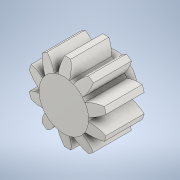
# Autodesk Inventor part: Spur Gear1
Saved by Autodesk Inventor 2022 (Build 260153000, 153)
## iProperties
CustomPartVersion: 1
Created: 2022-03-16
Part Number: Spur Gear1
Material: Steel
Document SubType Name: Modeling
Designer: zac-h
Categories: <?xml version="1.0" encoding="UTF-16"?> <MemberInstance><Categories><FamilyTemplate><FamilyTemplateParameter ValueType="xs:double" Id="1" ObjectReferenceKey="da_z" ObjectType="kUserParameterObject"/><FamilyTemplateParameter ValueType="xs:double" Id="2" ObjectReferenceKey="da_b" ObjectType="kUserParameterObject"/><FamilyTemplateParameter ValueType="xs:double" Id="3" ObjectReferenceKey="da_beta" ObjectType="kUserParameterObject"/><FamilyTemplateParameter ValueType="xs:double" Id="4" ObjectReferenceKey="da_da" ObjectType="kUserParameterObject"/><FamilyTemplateParameter ValueType="xs:double" Id="5" ObjectReferenceKey="da_aw" ObjectType="kUserParameterObject"/><FamilyTemplateParameter ValueType="xs:string" Id="6" ObjectReferenceKey="EAIAABAAAAC/AAAAAAAAAIAAAAAAAAAA" ObjectType="83910656" SubObjectId="SurfaceGeometry"/></FamilyTemplate><ParamToTemplateMap><ParamToTemplate CategoryParameter="//CategoryParameter[@InternalName='046C89C9-8512-4d59-83FE-43B91F4F132A']" TemplateParameter="1"/><ParamToTemplate CategoryParameter="//CategoryParameter[@InternalName='2552DF32-E462-4b46-AEBF-C6C7768E72AC']" TemplateParameter="2"/><ParamToTemplate CategoryParameter="//CategoryParameter[@InternalName='C9EE641D-15FC-4fae-A226-E94C4372FDD7']" TemplateParameter="3"/><ParamToTemplate><ParamToTemplate CategoryParameter="//CategoryParameter[@InternalName='00B6519A-459B-49c7-AD84-2E56D39A5744']" ConstantValue="0.000000"/></ParamToTemplate><ParamToTemplate><ParamToTemplate CategoryParameter="//CategoryParameter[@InternalName='04B31F0E-C7A6-4894-AA32-9629BEFACF47']" ConstantValue="1.000000"/></ParamToTemplate><ParamToTemplate><ParamToTemplate CategoryParameter="//CategoryParameter[@InternalName='43CBEC2E-7847-49e7-A936-2F7889FCB2D9']" ConstantValue="0.250000"/></ParamToTemplate><ParamToTemplate><ParamToTemplate CategoryParameter="//CategoryParameter[@InternalName='B1EFC894-105D-4ebd-86BF-FA20ED196853']" ConstantValue="0.333500"/></ParamToTemplate><ParamToTemplate><ParamToTemplate CategoryParameter="//CategoryParameter[@InternalName='51175063-3D10-4879-93E8-6246FE8B403D']" ConstantValue="2061532430.657340"/></ParamToTemplate><ParamToTemplate><ParamToTemplate CategoryParameter="//CategoryParameter[@InternalName='A3A52E27-4454-46a9-B0BD-C932399B70AF']" ConstantValue="0.300000"/></ParamToTemplate><ParamToTemplate><ParamToTemplate CategoryParameter="//CategoryParameter[@InternalName='91B76062-C214-41d9-B1B9-14D2AB99603D']" ConstantValue="0.100000"/></ParamToTemplate><ParamToTemplate><ParamToTemplate CategoryParameter="//CategoryParameter[@InternalName='374E806E-8B8A-4dda-A9AA-1039D6500AD2']" ConstantValue="10.000000"/></ParamToTemplate><ParamToTemplate><ParamToTemplate CategoryParameter="//CategoryParameter[@InternalName='2D373A89-B862-43d6-8D0B-0CBF12AB9F6C']" ConstantValue="0.253073"/></ParamToTemplate><ParamToTemplate CategoryParameter="//CategoryParameter[@InternalName='37777632-D6A2-4fac-9D53-DB8ACD95C989']" TemplateParameter="4"/><ParamToTemplate CategoryParameter="//CategoryParameter[@InternalName='FD1017F1-B727-4f7e-9707-0F86F1FF9423']" TemplateParameter="5"/><ParamToTemplate><ParamToTemplate CategoryParameter="//CategoryParameter[@InternalName='9E1B4470-B2D3-4ff1-B813-535BB4CDF51A']" ConstantValue="3523220.976809"/></ParamToTemplate><ParamToTemplate><ParamToTemplate CategoryParameter="//CategoryParameter[@InternalName='F8452263-BFF6-458c-9FB1-07C4B99E95CD']" ConstantValue="11397033.805607"/></ParamToTemplate><ParamToTemplate><ParamToTemplate CategoryParameter="//CategoryParameter[@InternalName='3E3BB259-FD49-497f-8171-6EBC954A3479']" ConstantValue="2.000000"/></ParamToTemplate><ParamToTemplate CategoryParameter="//CategoryParameter[@InternalName='27C3BAF2-7550-4e4b-AE2C-0DB134B7D9B7']" TemplateParameter="6"/></ParamToTemplateMap><Category DisplayName="Gear" InternalName="DC85795E-93AB-48d5-8EEE-5A27447B64BD" Mnemonic="Gear"><CategoryParameter DisplayName="z" InternalName="046C89C9-8512-4d59-83FE-43B91F4F132A" Mnemonic="z"/><CategoryParameter DisplayName="b" InternalName="2552DF32-E462-4b46-AEBF-C6C7768E72AC" Mnemonic="b"/><CategoryParameter DisplayName="||b|" InternalName="C9EE641D-15FC-4fae-A226-E94C4372FDD7" Mnemonic="beta"/><CategoryParameter DisplayName="x" InternalName="00B6519A-459B-49c7-AD84-2E56D39A5744" Mnemonic="x"/><CategoryParameter DisplayName="a*" InternalName="04B31F0E-C7A6-4894-AA32-9629BEFACF47" Mnemonic="a"/><CategoryParameter DisplayName="c*" InternalName="43CBEC2E-7847-49e7-A936-2F7889FCB2D9" Mnemonic="c"/><CategoryParameter DisplayName="r|.f|*" InternalName="B1EFC894-105D-4ebd-86BF-FA20ED196853" Mnemonic="rf"/><CategoryParameter DisplayName="E" InternalName="51175063-3D10-4879-93E8-6246FE8B403D" Mnemonic="E"/><CategoryParameter DisplayName="||m|" InternalName="A3A52E27-4454-46a9-B0BD-C932399B70AF" Mnemonic="mi"/><Category DisplayName="SpurGear" InternalName="26C5A22E-A91E-4dfd-A3B3-23CCAFAE1764" Mnemonic="SpurGear"><CategoryParameter DisplayName="m" InternalName="91B76062-C214-41d9-B1B9-14D2AB99603D" Mnemonic="m"/><CategoryParameter DisplayName="P" InternalName="374E806E-8B8A-4dda-A9AA-1039D6500AD2" Mnemonic="PP"/><CategoryParameter DisplayName="||a|" InternalName="2D373A89-B862-43d6-8D0B-0CBF12AB9F6C" Mnemonic="alpha"/><CategoryParameter DisplayName="d|.a|" InternalName="37777632-D6A2-4fac-9D53-DB8ACD95C989" Mnemonic="da"/><CategoryParameter DisplayName="a|.w|" InternalName="FD1017F1-B727-4f7e-9707-0F86F1FF9423" Mnemonic="aw"/><CategoryParameter DisplayName="||s||.Flim|" InternalName="9E1B4470-B2D3-4ff1-B813-535BB4CDF51A" Mnemonic="sFlim"/><CategoryParameter DisplayName="||s||.Hlim|" InternalName="F8452263-BFF6-458c-9FB1-07C4B99E95CD" Mnemonic="sHlim"/><CategoryParameter DisplayName="type" InternalName="3E3BB259-FD49-497f-8171-6EBC954A3479" Mnemonic="type"/><CategoryParameter DisplayName="PitchDiameter" InternalName="27C3BAF2-7550-4e4b-AE2C-0DB134B7D9B7" Mnemonic="IDS_PITCHDIAM"/></Category></Category></Categories></MemberInstance>
Density: 1 g/cm^3
Appearance: Steel
Author: zac-h
## iProperties of the stored document Spur Gear11_3DPrint.ipt
Created: 2022-03-19
Part Number: Spur Gear11_3DPrint
Material: Generic
Document SubType Name: Modeling
Designer: zac-h
Density: 1 g/cm^3
Appearance: Default
Author: zac-h
Autodesk Inventor part; units mm, degrees
ref_plane "YZ Plane" through (0, 0, 0) normal (1, 0, 0) x (0, 1, 0)
ref_plane "XZ Plane" through (0, 0, 0) normal (0, 1, 0) x (-1, 0, 0)
ref_plane "XY Plane" through (0, 0, 0) normal (0, 0, 1) x (1, 0, 0)
sketch "Sketch1" plane through (0, 0, 0) normal (0, 0, 1) x (1, 0, 0)
  circle A0 centre (0, 0) radius 5.9807
  dimension "d0" = 11.9613
  constraints: 1 centre point
  measures "d0" diameter of A0
extrude "Extrusion1" add sketch "Sketch1" along normal blind 6.35
sketch "Sketch2" plane through (0, 0, 0) normal (0, 0, -1) x (-1, 0, 0)
  circle A0 centre (0, 0) radius 5.9807 projected
  circle A1 centre (0, 0) radius 5
  dimension "d3" = 10
  constraints: 1 centre point, 1 coincident
  measures "d3" diameter of A1
surface extrude "Pitch Diameter" sketch "Sketch2" against normal through all shown no curves A1
ref_plane "Work Plane1" through (0, 0, 0) normal (1, 0, 0) x (0, 1, 0)
ref_plane "Work Plane2" through (0, 0, 0) normal (0.9510565, 0.309017, 0) x (0, 0, 1)
ref_plane "Work Plane3" through (0, 0, 3.175) normal (0, 0, -1) x (-1, 0, 0)
spur gear teeth "Spur Gear" teeth 10 pitch diameter 10 tip diameter 11.9613 root diameter 7.5 face width 6.35 start plane through (0, 0, 0) normal (0, 0, -1) x (-1, 0, 0)
sketch "Sketch3" plane through (0, 0, 6.35) normal (0, 0, 1) x (1, 0, 0)
  line L0 (1.6625, 1.6625) -> (-1.6625, 1.6625)
  line L1 (-1.6625, 1.6625) -> (-1.6625, -1.6625)
  line L2 (-1.6625, -1.6625) -> (1.6625, -1.6625)
  line L3 (1.6625, -1.6625) -> (1.6625, 1.6625)
  line L4 (1.6625, 1.6625) -> (-1.6625, -1.6625) construction
  line L5 (-1.6625, 1.6625) -> (1.6625, -1.6625) construction
  point P0 (0, 0)
  dimension "d20" = 3.325
  constraints: 12 end point, 2 midpoint, 2 parallel, 2 perpendicular, 1 horizontal
  measures "d20" distance of L2.end L1.end
extrude "Extrusion2" cut sketch "Sketch3" against normal through all
sketch "Sketch4" plane through (0, 0, 0) normal (0, 0, -1) x (-1, 0, 0)
  line L0 (1.6625, -1.6625) -> (-1.6625, -1.6625) projected
  line L1 (-1.6625, -1.6625) -> (-1.6625, 1.6625) projected
  line L2 (-1.6625, 1.6625) -> (1.6625, 1.6625) projected
  line L3 (1.6625, 1.6625) -> (1.6625, -1.6625) projected
  arc A0 (2.8515, 2.4354) -> (3.8841, 4.5477) centre (-1.3922, 5.8185) ccw projected
  arc A1 (3.8841, 4.5477) -> (3.1249, 5.0993) centre (0, 0) ccw projected
  arc A2 (3.1249, 5.0993) -> (1.4351, 3.4645) centre (5.9639, 0.474) ccw projected
  arc A3 (1.4351, 3.4645) -> (0.8754, 3.6464) centre (0, 0) ccw projected
  arc A4 (0.8754, 3.6464) -> (0.4692, 5.9622) centre (-4.5463, 3.889) ccw projected
  arc A5 (0.4692, 5.9622) -> (-0.4692, 5.9622) centre (0, 0) ccw projected
  arc A6 (-0.4692, 5.9622) -> (-0.8754, 3.6464) centre (4.5463, 3.889) ccw projected
  arc A7 (-0.8754, 3.6464) -> (-1.4351, 3.4645) centre (0, 0) ccw projected
  arc A8 (-1.4351, 3.4645) -> (-3.1249, 5.0993) centre (-5.9639, 0.474) ccw projected
  arc A9 (-3.1249, 5.0993) -> (-3.8841, 4.5477) centre (0, 0) ccw projected
  arc A10 (-3.8841, 4.5477) -> (-2.8515, 2.4354) centre (1.3922, 5.8185) ccw projected
  arc A11 (-2.8515, 2.4354) -> (-3.1974, 1.9594) centre (0, 0) ccw projected
  arc A12 (-3.1974, 1.9594) -> (-5.5254, 2.2887) centre (-5.1035, -3.1221) ccw projected
  arc A13 (-5.5254, 2.2887) -> (-5.8154, 1.3962) centre (0, 0) ccw projected
  arc A14 (-5.8154, 1.3962) -> (-3.7384, 0.2942) centre (-2.2937, 5.5256) ccw projected
  arc A15 (-3.7384, 0.2942) -> (-3.7384, -0.2942) centre (0, 0) ccw projected
  arc A16 (-3.7384, -0.2942) -> (-5.8154, -1.3962) centre (-2.2937, -5.5256) ccw projected
  arc A17 (-5.8154, -1.3962) -> (-5.5254, -2.2887) centre (0, 0) ccw projected
  arc A18 (-5.5254, -2.2887) -> (-3.1974, -1.9594) centre (-5.1035, 3.1221) ccw projected
  arc A19 (-3.1974, -1.9594) -> (-2.8515, -2.4354) centre (0, 0) ccw projected
  arc A20 (-2.8515, -2.4354) -> (-3.8841, -4.5477) centre (1.3922, -5.8185) ccw projected
  arc A21 (-3.8841, -4.5477) -> (-3.1249, -5.0993) centre (0, 0) ccw projected
  arc A22 (-3.1249, -5.0993) -> (-1.4351, -3.4645) centre (-5.9639, -0.474) ccw projected
  arc A23 (-1.4351, -3.4645) -> (-0.8754, -3.6464) centre (0, 0) ccw projected
  arc A24 (-0.8754, -3.6464) -> (-0.4692, -5.9622) centre (4.5463, -3.889) ccw projected
  arc A25 (-0.4692, -5.9622) -> (0.4692, -5.9622) centre (0, 0) ccw projected
  arc A26 (0.4692, -5.9622) -> (0.8754, -3.6464) centre (-4.5463, -3.889) ccw projected
  arc A27 (0.8754, -3.6464) -> (1.4351, -3.4645) centre (0, 0) ccw projected
  arc A28 (1.4351, -3.4645) -> (3.1249, -5.0993) centre (5.9639, -0.474) ccw projected
  arc A29 (3.1249, -5.0993) -> (3.8841, -4.5477) centre (0, 0) ccw projected
  arc A30 (3.8841, -4.5477) -> (2.8515, -2.4354) centre (-1.3922, -5.8185) ccw projected
  arc A31 (2.8515, -2.4354) -> (3.1974, -1.9594) centre (0, 0) ccw projected
  arc A32 (3.1974, -1.9594) -> (5.5254, -2.2887) centre (5.1035, 3.1221) ccw projected
  arc A33 (5.5254, -2.2887) -> (5.8154, -1.3962) centre (0, 0) ccw projected
  arc A34 (5.8154, -1.3962) -> (3.7384, -0.2942) centre (2.2937, -5.5256) ccw projected
  arc A35 (3.7384, -0.2942) -> (3.7384, 0.2942) centre (0, 0) ccw projected
  arc A36 (3.7384, 0.2942) -> (5.8154, 1.3962) centre (2.2937, 5.5256) ccw projected
  arc A37 (5.8154, 1.3962) -> (5.5254, 2.2887) centre (0, 0) ccw projected
  arc A38 (5.5254, 2.2887) -> (3.1974, 1.9594) centre (5.1035, -3.1221) ccw projected
  arc A39 (3.1974, 1.9594) -> (2.8515, 2.4354) centre (0, 0) ccw projected
  circle A40 centre (0, 0) radius 3.175
  dimension "d23" = 6.35
  constraints: 1 centre point, 1 coincident
  measures "d23" diameter of A40
extrude "Extrusion3" add sketch "Sketch4" along normal blind 1.5875 contours A40
sketch "Sketch5" plane through (0, 0, 0) normal (0, 1, 0) x (-1, 0, 0)
  line L0 (3.75, 6.35) -> (3.7384, 6.35) projected
  line L1 (3.75, 6.35) -> (6.7127, 5.5561)
  line L2 (3.75, 6.35) -> (6.8173, 6.35) construction
  line L3 (6.7127, 5.5561) -> (6.7127, 6.35)
  line L4 (5.8154, 6.35) -> (3.7384, 6.35) projected
  line L5 (6.7127, 6.35) -> (3.7384, 6.35)
  line L6 (0, 6.2413) -> (0, 0) construction
  dimension "d26" = 15
  constraints: 10 end point, 2 perpendicular, 1 coincident, 1 equal length, 1 horizontal, 1 vertical
  measures "d26" angle of L1 L2
revolve "Revolution1" cut sketch "Sketch5" angle 360 about axis through (0, 0, 6.2413) along (0, 0, -1)
sketch "Sketch6" plane through (0, 0, 6.35) normal (0, 0, 1) x (1, 0, 0)
  line L0 (1.6625, -1.6625) -> (-1.6625, -1.6625) projected
  line L1 (-1.6625, -1.6625) -> (-1.6625, 1.6625) projected
  line L2 (-1.6625, 1.6625) -> (1.6625, 1.6625) projected
  line L3 (1.6625, 1.6625) -> (1.6625, -1.6625) projected
  arc A0 (-0.8754, -3.6464) -> (0.8754, -3.6464) centre (0, 0) ccw projected
  arc A1 (0.8754, -3.6464) -> (1.4351, -3.4645) centre (0, 0) ccw projected
  arc A2 (1.4351, -3.4645) -> (2.8515, -2.4354) centre (0, 0) ccw projected
  arc A3 (2.8515, -2.4354) -> (3.1974, -1.9594) centre (0, 0) ccw projected
  arc A4 (3.1974, -1.9594) -> (3.7384, -0.2942) centre (0, 0) ccw projected
  arc A5 (3.7384, -0.2942) -> (3.7384, 0.2942) centre (0, 0) ccw projected
  arc A6 (3.7384, 0.2942) -> (3.1974, 1.9594) centre (0, 0) ccw projected
  arc A7 (3.1974, 1.9594) -> (2.8515, 2.4354) centre (0, 0) ccw projected
  arc A8 (2.8515, 2.4354) -> (1.4351, 3.4645) centre (0, 0) ccw projected
  arc A9 (1.4351, 3.4645) -> (0.8754, 3.6464) centre (0, 0) ccw projected
  arc A10 (0.8754, 3.6464) -> (-0.8754, 3.6464) centre (0, 0) ccw projected
  arc A11 (-0.8754, 3.6464) -> (-1.4351, 3.4645) centre (0, 0) ccw projected
  arc A12 (-1.4351, 3.4645) -> (-2.8515, 2.4354) centre (0, 0) ccw projected
  arc A13 (-2.8515, 2.4354) -> (-3.1974, 1.9594) centre (0, 0) ccw projected
  arc A14 (-3.1974, 1.9594) -> (-3.7384, 0.2942) centre (0, 0) ccw projected
  arc A15 (-3.7384, 0.2942) -> (-3.7384, -0.2942) centre (0, 0) ccw projected
  arc A16 (-3.7384, -0.2942) -> (-3.1974, -1.9594) centre (0, 0) ccw projected
  arc A17 (-3.1974, -1.9594) -> (-2.8515, -2.4354) centre (0, 0) ccw projected
  arc A18 (-2.8515, -2.4354) -> (-1.4351, -3.4645) centre (0, 0) ccw projected
  arc A19 (-1.4351, -3.4645) -> (-0.8754, -3.6464) centre (0, 0) ccw projected
extrude "Extrusion4" add sketch "Sketch6" against normal blind 2 contours L0 L1 L2 L3
equation "\"d0\" = da_da"
equation "\"d1\" = da_b"
equation "\"d3\" = da_d"
equation "\"d15\" = da_aw"
equation "\"d19\" = da_aw"
equation "\"da_da\" = 11.961303"
equation "\"da_b\" = 6.35"
equation "\"da_d\" = 10"
equation "\"da_aw\" = 23.75408"
body "Solid1"
body "Srf1"
